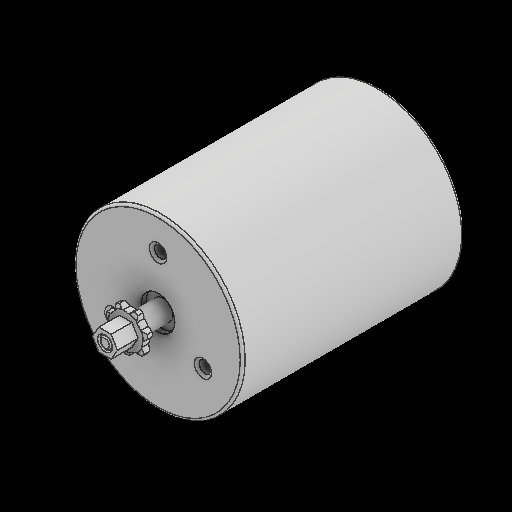
# Autodesk Inventor part: MY6812-12VDC-120W
Saved by Autodesk Inventor 2025.2 (Build 292293000, 293)
## iProperties
Created: 2025-10-04
Part Number: MY6812-12VDC-120W
Material: Generic
Document SubType Name: Modeling
Designer: valer
Density: 1 g/cm^3
Appearance: Default
Author: valer
Autodesk Inventor part; units mm, degrees
sketch "Base" plane through (0, 0, 0) normal (0, 0, 1) x (1, 0, 0)
  circle A0 centre (0, 0) radius 34
  dimension "d0" = 68
  constraints: 1 centre point, 1 coincident
  measures "d0" diameter of A0
extrude "BaseFeature" add sketch "Base" along normal blind 89
sketch "Sketch2" plane through (0, 0, 0) normal (0, 0, -1) x (-1, 0, 0)
  circle A0 centre (0, 0) radius 14.75
  dimension "d3" = 29.5
  constraints: 1 centre point, 1 coincident
  measures "d3" diameter of A0
extrude "Extrusion2" add sketch "Sketch2" along normal blind 11
fillet "Fillet1" radius 1 3 edges at (14.75, 0, -11) (-34, 0, 0) (-34, 0, 89)
sketch "Sketch3" plane through (0, 0, 89) normal (0, 0, 1) x (1, 0, 0)
  circle A0 centre (0, 0) radius 34 projected
  circle A1 centre (0, 0) radius 6.75
  dimension "d7" = 13.5
  constraints: 1 centre point, 1 coincident
  measures "d7" diameter of A1
extrude "Extrusion3" cut sketch "Sketch3" against normal blind 2 contours A1
sketch "Sketch4" plane through (0, 0, 87) normal (0, 0, 1) x (1, 0, 0)
  circle A0 centre (0, 0) radius 4
  dimension "d10" = 8
  constraints: 1 centre point, 1 coincident
  measures "d10" diameter of A0
ref_plane "Work Plane1" through (0, 0, 99) normal (0, 0, 1) x (1, 0, 0)
extrude "Extrusion4" add sketch "Sketch4" along normal up to surface (12 mm away)
sketch "Sketch5" plane through (0, 0, 99) normal (0, 0, 1) x (1, 0, 0)
  circle A0 centre (0, 0) radius 33 construction
  circle A1 centre (0, 0) radius 8.5 construction
  circle A2 centre (0, 0) radius 4 construction
  line L0 (0, 0) -> (0, -8.5) construction
  line L1 (-0.75, -8.5) -> (0.75, -8.5)
  circle A3 centre (0, 0) radius 6.75 projected
  line L2 (-0.75, -8.5) -> (-1.75, -6.5192)
  line L3 (-47.6, 0) -> (47.6, 0) construction
  line L4 (0.75, -8.5) -> (1.75, -6.5192)
  line L5 (7.1132, -4.7133) -> (6.188, -2.6965)
  line L6 (6.178, -5.886) -> (4.0058, -5.4329)
  line L7 (6.178, -5.886) -> (7.1132, -4.7133)
  line L8 (8.12, 2.6226) -> (5.9663, 3.1568)
  line L9 (8.4538, 1.1602) -> (6.7452, -0.2555)
  line L10 (8.4538, 1.1602) -> (8.12, 2.6226)
  line L11 (3.0123, 7.9836) -> (1.2519, 6.6329)
  line L12 (4.3637, 7.3328) -> (4.4053, 5.1143)
  line L13 (4.3637, 7.3328) -> (3.0123, 7.9836)
  line L14 (-4.3637, 7.3328) -> (-4.4053, 5.1143)
  line L15 (-3.0123, 7.9836) -> (-1.2519, 6.6329)
  line L16 (-3.0123, 7.9836) -> (-4.3637, 7.3328)
  line L17 (-8.4538, 1.1602) -> (-6.7452, -0.2555)
  line L18 (-8.12, 2.6226) -> (-5.9663, 3.1568)
  line L19 (-8.12, 2.6226) -> (-8.4538, 1.1602)
  line L20 (-6.178, -5.886) -> (-4.0058, -5.4329)
  line L21 (-7.1132, -4.7133) -> (-6.188, -2.6965)
  line L22 (-7.1132, -4.7133) -> (-6.178, -5.886)
  point P0 (6.6456, -5.2997)
  point P1 (8.2869, 1.8914)
  point P2 (3.688, 7.6582)
  point P3 (-3.688, 7.6582)
  point P4 (-8.2869, 1.8914)
  point P5 (-6.6456, -5.2997)
  dimension "d14" = 17
  dimension "d23" = 1.5
  dimension "d24" = 3.5
  dimension "d27" = 360
  constraints: 44 end point, 2 perpendicular, 1 coincident, 1 midpoint, 1 symmetric about line, 1 vertical alignment, 61 other
  measures "d23" distance of L1.end L1.start
  measures "d24" distance of L4.end L2.end
extrude "Extrusion5" add sketch "Sketch5" along normal blind 3 separate body
sketch "Sketch6" plane through (0, 0, 102) normal (0, 0, 1) x (1, 0, 0)
  line L0 (-2.5, 4.3301) -> (2.5, 4.3301)
  line L1 (2.5, 4.3301) -> (5, 0)
  line L2 (5, 0) -> (2.5, -4.3301)
  line L3 (2.5, -4.3301) -> (-2.5, -4.3301)
  line L4 (-2.5, -4.3301) -> (-5, 0)
  line L5 (-5, 0) -> (-2.5, 4.3301)
  line L6 (-47.6, 0) -> (47.6, 0) construction
  point P0 (0, 0)
  point P1 (0, 0)
  point P2 (0, 0)
  dimension "d17" = 10
  constraints: 12 end point, 1 coincident, 1 point on line, 13 other
  measures "d17" distance of L1.end L4.end
extrude "Extrusion6" add sketch "Sketch6" along normal blind 8.33 bodies 1
sketch "Sketch7" plane through (0, 0, 110.33) normal (0, 0, 1) x (1, 0, 0)
  circle A0 centre (0, 0) radius 2.5
  dimension "d29" = 5
  constraints: 1 centre point, 1 coincident
  measures "d29" diameter of A0
extrude "Extrusion7" cut sketch "Sketch7" against normal blind 1 bodies 1
chamfer "Chamfer1" distance 0.5 angle 45 1 edges at (-2.5, 0, 110.33)
sketch "Sketch8" plane through (0, 0, 109.33) normal (0, 0, 1) x (1, 0, 0)
  circle A0 centre (0, 0) radius 2.25
  dimension "d36" = 4.5
  constraints: 1 centre point, 1 coincident
  measures "d36" diameter of A0
extrude "Extrusion8" add sketch "Sketch8" along normal blind 1 bodies 1
fillet "Fillet3" radius 0.5 1 edges at (-2.25, 0, 110.33)
sketch "Sketch9" plane through (0, 0, 0) normal (1, 0, 0) x (0, 1, 0)
  line L0 (-8.5, 99) -> (-8.5, 102) construction
  line L1 (-8.5, 100.5) -> (7.9836, 100.5) construction
  line L2 (7.9836, 99) -> (7.9836, 102) construction
  line L3 (-8.5, 102) -> (7.9836, 102)
  line L4 (-8.5, 99) -> (7.9836, 99)
  line L5 (-8.5, 101.5) -> (-8.5, 99.5)
  line L6 (0, 102) -> (0, 110.33) projected
  line L7 (0, 102) -> (0, 99)
  line L8 (-8.5, 101.5) -> (-7, 102)
  line L9 (-7, 102) -> (-7, 100.5) construction
  line L10 (-8.5, 102) -> (-6.5192, 102) projected
  line L11 (-8.5, 99) -> (-8.5, 102) projected
  line L12 (-8.5, 99.5) -> (-7, 99)
  point P0 (0, 0)
  dimension "d40" = 2
  dimension "d41" = 1.5
  constraints: 16 end point, 4 midpoint, 3 point on line, 2 perpendicular, 1 horizontal, 1 parallel, 1 symmetric about line, 1 vertical
  measures "d40" distance of L5.start L5.end
  measures "d41" distance between parallel lines of L9 L5
revolve "Revolution1" add sketch "Sketch9" angle 360 about axis through (0, 0, 102) along (0, 0, -1) separate body contours L3 L7 L4 L12 L5 L8
combine bodies "Combine1" operation type common bodies to combine 2 3
sketch "Sketch10" plane through (0, 0, 89) normal (0, 0, 1) x (1, 0, 0)
  circle A0 centre (0, 0) radius 6.75 construction
  line L0 (0, -47.6) -> (0, 47.6) construction
  line L1 (0, 20.7846) -> (18, -10.3923) construction
  line L2 (18, -10.3923) -> (-18, -10.3923) construction
  line L3 (-18, -10.3923) -> (0, 20.7846) construction
  circle A1 centre (0, 20.7846) radius 2.5
  circle A2 centre (18, -10.3923) radius 2.5
  circle A3 centre (-18, -10.3923) radius 2.5
  dimension "d43" = 36
  dimension "d44" = 5
  constraints: 6 end point, 4 coincident, 3 centre point, 2 equal radius, 1 point on line, 7 other
  measures "d43" distance of L1.start L1.end
  measures "d44" diameter of A1
extrude "Extrusion9" cut sketch "Sketch10" against normal blind 10 bodies 1
fillet "Fillet4" radius 1 3 edges at (-2.5, 20.7846, 89) (-20.5, -10.3923, 89) (15.5, -10.3923, 89)
ref_plane "MidPlane" through (0, 0, 44.5) normal (0, 0, -1) x (-1, 0, 0)
ref_plane "SprocketMidPlane" through (0, 0, 100.5) normal (0, 0, 1) x (1, 0, 0)
body "Solid1"
body "Solid3"
